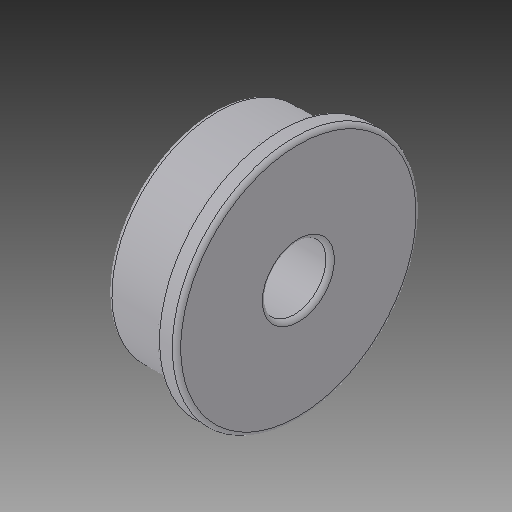
# Autodesk Inventor part: Roulement a bille F623ZZ
Saved by Autodesk Inventor 2017 (Build 210142000, 142)
## iProperties
Company: FABLAB Frenchmakers
Part Number: Roulement a bille F623ZZ
Material: ----------
Document SubType Name: Modeling
Designer: FABLAB Frenchmakers
Density: 7.86 g/cm^3
Appearance: Métal - Acier
Mass: 2.44003 g
Surface Area: 3.48462 cm^2
Volume: 0.310437 cm^3
Stock Number: 1420-01-06
Project: 1420 Vauban 3D XL
Catalog Web Link: http://frenchmakers.com/
Autodesk Inventor part; units mm, degrees
ref_plane "YZ Plane" through (0, 0, 0) normal (1, 0, 0) x (0, 1, 0)
ref_plane "XZ Plane" through (0, 0, 0) normal (0, 1, 0) x (-1, 0, 0)
ref_plane "XY Plane" through (0, 0, 0) normal (0, 0, 1) x (1, 0, 0)
sketch "Esquisse1" plane through (0, 0, 0) normal (0, 0, 1) x (1, 0, 0)
  line L0 (-4.4077, 0) -> (0, 0)
  line L1 (1.8, 1.5) -> (-1.8, 1.5)
  line L2 (-2, 1.7) -> (-2, 4.8)
  line L3 (-1.8, 5) -> (0.8, 5)
  line L4 (1, 5.2) -> (1, 5.55)
  line L5 (1.2, 5.75) -> (1.8, 5.75)
  line L6 (2, 5.55) -> (2, 1.7)
  arc A0 (-1.8, 5) -> (-2, 4.8) centre (-1.8, 4.8) ccw
  arc A1 (-2, 1.7) -> (-1.8, 1.5) centre (-1.8, 1.7) ccw
  arc A2 (1.8, 1.5) -> (2, 1.7) centre (1.8, 1.7) ccw
  arc A3 (2, 5.55) -> (1.8, 5.75) centre (1.8, 5.55) ccw
  arc A4 (1.2, 5.75) -> (1, 5.55) centre (1.2, 5.55) ccw
  arc A5 (0.8, 5) -> (1, 5.2) centre (0.8, 5.2) ccw
  point P0 (1, 5.75)
  point P1 (2, 5.75)
  dimension "d0" = 3
  dimension "d1" = 4
  dimension "d2" = 11.5
  dimension "d3" = 10
  dimension "d4" = 1
  dimension "d5" = 2
  dimension "d6" = 0.2
  constraints: 14 end point, 12 point on circle, 12 tangent, 6 centre point, 5 equal radius, 5 perpendicular, 4 point on line, 2 horizontal, 1 coincident
  measures "d0" diameter of L1 L0
  measures "d1" distance between parallel lines of L6 L2
  measures "d2" diameter of L5 L0
  measures "d3" diameter of L3 L0
  measures "d4" distance of point (1, 5.75) point (2, 5.75)
  measures "d5" distance from line of L6 point (0, 0)
  measures "d6" radius of A0
revolve "Révolution1" add sketch "Esquisse1" angle 360 about axis through (-4.4077, 0, 0) along (1, 0, 0)
equation "\"d5\" = 0.5 * d1"
